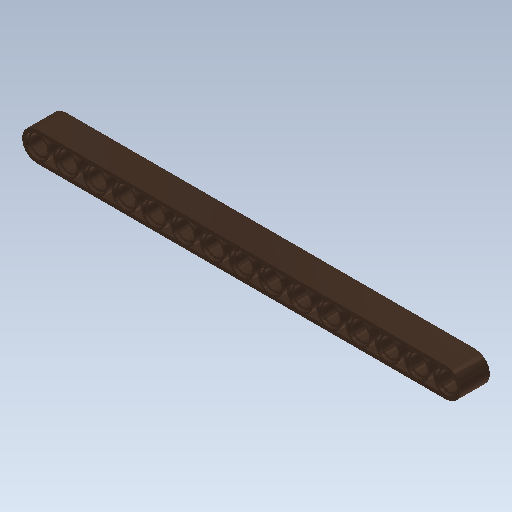
# Autodesk Inventor part: 15M Beam
Saved by Autodesk Inventor 2020 (Build 240168000, 168)
## iProperties
Created: 2014-02-10
Part Number: 15M Beam
Document SubType Name: Modeling
Designer: jleonard
Density: 8.87 g/cm^3
Material: Bronze, Cast
Appearance: Bronze - Satin
Author: jleonard
Autodesk Inventor part; units mm, degrees
ref_plane "YZ Plane" through (0, 0, 0) normal (1, 0, 0) x (0, 1, 0)
ref_plane "XZ Plane" through (0, 0, 0) normal (0, 1, 0) x (-1, 0, 0)
ref_plane "XY Plane" through (0, 0, 0) normal (0, 0, 1) x (1, 0, 0)
sketch "Sketch2" plane through (0, 0, 0) normal (0, 0, 1) x (1, 0, 0)
  arc A0 (-56, 4) -> (-56, -4) centre (-56, 0) ccw
  arc A1 (56, -4) -> (56, 4) centre (56, 0) ccw
  line L0 (-56, 4) -> (56, 4)
  line L1 (-56, -4) -> (56, -4)
  line L2 (-84, 0) -> (84, 0) projected
  line L3 (0, -5.6) -> (0, 5.6) projected
  point P0 (0, 0)
  dimension "d0" = 4
  dimension "d1" = 4
  dimension "d2" = 112
  dimension "d3" = 0
  dimension "d4" = 56
  dimension "d9" = 180
  dimension "d10" = 0
  dimension "d268" = 112
  constraints: 6 point on circle, 4 end point, 2 centre point, 2 point on line, 2 tangent
  measures "d0" radius of A0
  measures "d1" radius of A1
  measures "d2" distance of A1.centre A0.centre
  measures "d3" distance from line of A0.centre L2
  measures "d4" distance from line of A0.centre L3
  measures "d9" angle of L0 L2
  measures "d10" distance from line of L2 A1.centre
  measures "d268" distance of L1.start L1.end
extrude "Extrusion1" add sketch "Sketch2" along normal blind 8
sketch "Sketch27" plane through (0, 0, 8) normal (0, 0, 1) x (1, 0, 0)
  arc A0 (-56, 4) -> (-56, -4) centre (-56, 0) ccw projected
  circle A1 centre (-56, 0) radius 2.5
  line L0 (-84, 0) -> (84, 0) projected
  circle A2 centre (-48, 0) radius 2.5
  circle A3 centre (-40, 0) radius 2.5
  circle A4 centre (-32, 0) radius 2.5
  circle A5 centre (-24, 0) radius 2.5
  circle A6 centre (-16, 0) radius 2.5
  circle A7 centre (-8, 0) radius 2.5
  circle A8 centre (0, 0) radius 2.5
  circle A9 centre (8, 0) radius 2.5
  circle A10 centre (16, 0) radius 2.5
  circle A11 centre (24, 0) radius 2.5
  circle A12 centre (32, 0) radius 2.5
  circle A13 centre (40, 0) radius 2.5
  circle A14 centre (48, 0) radius 2.5
  circle A15 centre (56, 0) radius 2.5
  dimension "d269" = 5
  dimension "d275" = 8
  constraints: 15 centre point, 1 coincident, 1 horizontal, 28 other
  measures "d269" diameter of A1
  measures "d275" distance of A1.centre A2.centre
extrude "Extrusion26" cut sketch "Sketch27" against normal through all
sketch "Sketch28" plane through (0, 0, 8) normal (0, 0, 1) x (1, 0, 0)
  circle A0 centre (56, 0) radius 2.5 projected
  circle A1 centre (48, 0) radius 2.5 projected
  circle A2 centre (40, 0) radius 2.5 projected
  circle A3 centre (32, 0) radius 2.5 projected
  circle A4 centre (24, 0) radius 2.5 projected
  circle A5 centre (16, 0) radius 2.5 projected
  circle A6 centre (8, 0) radius 2.5 projected
  circle A7 centre (0, 0) radius 2.5 projected
  circle A8 centre (-8, 0) radius 2.5 projected
  circle A9 centre (-16, 0) radius 2.5 projected
  circle A10 centre (-24, 0) radius 2.5 projected
  circle A11 centre (-32, 0) radius 2.5 projected
  circle A12 centre (-40, 0) radius 2.5 projected
  circle A13 centre (-48, 0) radius 2.5 projected
  circle A14 centre (-56, 0) radius 2.5 projected
  arc A15 (-56, 4) -> (-56, -4) centre (-56, 0) ccw projected
  circle A16 centre (-56, 0) radius 3
  line L0 (-84, 0) -> (84, 0) projected
  circle A17 centre (-48, 0) radius 3
  circle A18 centre (-40, 0) radius 3
  circle A19 centre (-32, 0) radius 3
  circle A20 centre (-24, 0) radius 3
  circle A21 centre (-16, 0) radius 3
  circle A22 centre (-8, 0) radius 3
  circle A23 centre (0, 0) radius 3
  circle A24 centre (8, 0) radius 3
  circle A25 centre (16, 0) radius 3
  circle A26 centre (24, 0) radius 3
  circle A27 centre (32, 0) radius 3
  circle A28 centre (40, 0) radius 3
  circle A29 centre (48, 0) radius 3
  circle A30 centre (56, 0) radius 3
  dimension "d279" = 6
  dimension "d285" = 8
  constraints: 15 centre point, 1 coincident, 1 horizontal, 28 other
  measures "d279" diameter of A16
  measures "d285" distance of A16.centre A17.centre
extrude "Extrusion27" cut sketch "Sketch28" against normal blind 0.8 contours L0 A30 A0 | A0 L0 A30 | A16 L0 A14 | L0 A14 A16 | A17 L0 A13 | L0 A13 A17 | A18 L0 A12 | L0 A12 A18 | A19 L0 A11 | L0 A11 A19 | A20 L0 A10 | L0 A10 A20 | A21 L0 A9 | L0 A9 A21 | A22 L0 A8 | L0 A8 A22 | A23 L0 A7 | L0 A7 A23 | A24 L0 A6 | L0 A6 A24 | A25 L0 A5 | L0 A5 A25 | A26 L0 A4 | L0 A4 A26 | A27 L0 A3 | L0 A3 A27 | A28 L0 A2 | L0 A2 A28 | A29 L0 A1 | L0 A1 A29
sketch "Sketch29" plane through (0, 0, 0) normal (0, 0, -1) x (-1, 0, 0)
  circle A0 centre (-56, 0) radius 2.5 projected
  circle A1 centre (-48, 0) radius 2.5 projected
  circle A2 centre (-40, 0) radius 2.5 projected
  circle A3 centre (-32, 0) radius 2.5 projected
  circle A4 centre (-24, 0) radius 2.5 projected
  circle A5 centre (-16, 0) radius 2.5 projected
  circle A6 centre (-8, 0) radius 2.5 projected
  circle A7 centre (0, 0) radius 2.5 projected
  circle A8 centre (8, 0) radius 2.5 projected
  circle A9 centre (16, 0) radius 2.5 projected
  circle A10 centre (24, 0) radius 2.5 projected
  circle A11 centre (32, 0) radius 2.5 projected
  circle A12 centre (40, 0) radius 2.5 projected
  circle A13 centre (48, 0) radius 2.5 projected
  circle A14 centre (56, 0) radius 2.5 projected
  arc A15 (-56, 4) -> (-56, -4) centre (-56, 0) ccw projected
  circle A16 centre (-56, 0) radius 3
  line L0 (84, 0) -> (-84, 0) projected
  circle A17 centre (-48, 0) radius 3
  circle A18 centre (-40, 0) radius 3
  circle A19 centre (-32, 0) radius 3
  circle A20 centre (-24, 0) radius 3
  circle A21 centre (-16, 0) radius 3
  circle A22 centre (-8, 0) radius 3
  circle A23 centre (0, 0) radius 3
  circle A24 centre (8, 0) radius 3
  circle A25 centre (16, 0) radius 3
  circle A26 centre (24, 0) radius 3
  circle A27 centre (32, 0) radius 3
  circle A28 centre (40, 0) radius 3
  circle A29 centre (48, 0) radius 3
  circle A30 centre (56, 0) radius 3
  dimension "d289" = 6
  dimension "d295" = 8
  constraints: 15 centre point, 1 coincident, 1 horizontal, 28 other
  measures "d289" diameter of A16
  measures "d295" distance of A16.centre A17.centre
extrude "Extrusion28" cut sketch "Sketch29" against normal blind 0.8 contours L0 A16 A0 | A0 L0 A16 | A30 L0 A14 | L0 A14 A30 | A29 L0 A13 | L0 A13 A29 | A28 L0 A12 | L0 A12 A28 | A27 L0 A11 | L0 A11 A27 | A26 L0 A10 | L0 A10 A26 | A25 L0 A9 | L0 A9 A25 | A24 L0 A8 | L0 A8 A24 | A23 L0 A7 | L0 A7 A23 | A22 L0 A6 | L0 A6 A22 | A21 L0 A5 | L0 A5 A21 | A20 L0 A4 | L0 A4 A20 | A19 L0 A3 | L0 A3 A19 | A18 L0 A2 | L0 A2 A18 | A17 L0 A1 | L0 A1 A17
sketch "Sketch30" plane through (0, 0, 8) normal (0, 0, 1) x (1, 0, 0)
  circle A0 centre (-56, 0) radius 3 projected
  circle A1 centre (-48, 0) radius 3 projected
  arc A2 (-56, 4) -> (-56, -4) centre (-56, 0) ccw projected
  line L0 (-49.8028, 3) -> (-54.1972, 3)
  line L1 (-49.8028, -3) -> (-54.1972, -3)
  arc A3 (-54.1972, -3) -> (-54.1972, 3) centre (-56, 0) ccw
  arc A4 (-49.8028, 3) -> (-49.8028, -3) centre (-48, 0) ccw
  line L2 (-84, 0) -> (84, 0) projected
  line L3 (-41.8028, 3) -> (-46.1972, 3)
  line L4 (-41.8028, -3) -> (-46.1972, -3)
  arc A5 (-46.1972, -3) -> (-46.1972, 3) centre (-48, 0) ccw
  arc A6 (-41.8028, 3) -> (-41.8028, -3) centre (-40, 0) ccw
  line L5 (-33.8028, 3) -> (-38.1972, 3)
  line L6 (-33.8028, -3) -> (-38.1972, -3)
  arc A7 (-38.1972, -3) -> (-38.1972, 3) centre (-40, 0) ccw
  arc A8 (-33.8028, 3) -> (-33.8028, -3) centre (-32, 0) ccw
  line L7 (-25.8028, 3) -> (-30.1972, 3)
  line L8 (-25.8028, -3) -> (-30.1972, -3)
  arc A9 (-30.1972, -3) -> (-30.1972, 3) centre (-32, 0) ccw
  arc A10 (-25.8028, 3) -> (-25.8028, -3) centre (-24, 0) ccw
  line L9 (-17.8028, 3) -> (-22.1972, 3)
  line L10 (-17.8028, -3) -> (-22.1972, -3)
  arc A11 (-22.1972, -3) -> (-22.1972, 3) centre (-24, 0) ccw
  arc A12 (-17.8028, 3) -> (-17.8028, -3) centre (-16, 0) ccw
  line L11 (-9.8028, 3) -> (-14.1972, 3)
  line L12 (-9.8028, -3) -> (-14.1972, -3)
  arc A13 (-14.1972, -3) -> (-14.1972, 3) centre (-16, 0) ccw
  arc A14 (-9.8028, 3) -> (-9.8028, -3) centre (-8, 0) ccw
  line L13 (-1.8028, 3) -> (-6.1972, 3)
  line L14 (-1.8028, -3) -> (-6.1972, -3)
  arc A15 (-6.1972, -3) -> (-6.1972, 3) centre (-8, 0) ccw
  arc A16 (-1.8028, 3) -> (-1.8028, -3) centre (0, 0) ccw
  line L15 (6.1972, 3) -> (1.8028, 3)
  line L16 (6.1972, -3) -> (1.8028, -3)
  arc A17 (1.8028, -3) -> (1.8028, 3) centre (0, 0) ccw
  arc A18 (6.1972, 3) -> (6.1972, -3) centre (8, 0) ccw
  line L17 (14.1972, 3) -> (9.8028, 3)
  line L18 (14.1972, -3) -> (9.8028, -3)
  arc A19 (9.8028, -3) -> (9.8028, 3) centre (8, 0) ccw
  arc A20 (14.1972, 3) -> (14.1972, -3) centre (16, 0) ccw
  line L19 (22.1972, 3) -> (17.8028, 3)
  line L20 (22.1972, -3) -> (17.8028, -3)
  arc A21 (17.8028, -3) -> (17.8028, 3) centre (16, 0) ccw
  arc A22 (22.1972, 3) -> (22.1972, -3) centre (24, 0) ccw
  line L21 (30.1972, 3) -> (25.8028, 3)
  line L22 (30.1972, -3) -> (25.8028, -3)
  arc A23 (25.8028, -3) -> (25.8028, 3) centre (24, 0) ccw
  arc A24 (30.1972, 3) -> (30.1972, -3) centre (32, 0) ccw
  line L23 (38.1972, 3) -> (33.8028, 3)
  line L24 (38.1972, -3) -> (33.8028, -3)
  arc A25 (33.8028, -3) -> (33.8028, 3) centre (32, 0) ccw
  arc A26 (38.1972, 3) -> (38.1972, -3) centre (40, 0) ccw
  line L25 (46.1972, 3) -> (41.8028, 3)
  line L26 (46.1972, -3) -> (41.8028, -3)
  arc A27 (41.8028, -3) -> (41.8028, 3) centre (40, 0) ccw
  arc A28 (46.1972, 3) -> (46.1972, -3) centre (48, 0) ccw
  line L27 (54.1972, 3) -> (49.8028, 3)
  line L28 (54.1972, -3) -> (49.8028, -3)
  arc A29 (49.8028, -3) -> (49.8028, 3) centre (48, 0) ccw
  arc A30 (54.1972, 3) -> (54.1972, -3) centre (56, 0) ccw
  dimension "d299" = 7
  dimension "d300" = 7
  dimension "d306" = 8
  constraints: 56 end point, 56 point on circle, 28 centre point, 4 tangent, 2 coincident, 1 horizontal, 130 other
  measures "d299" diameter of A3
  measures "d300" diameter of A4
  measures "d306" distance of L0.start L3.start
extrude "Extrusion29" cut sketch "Sketch30" against normal through all contours A29 L27 A30 L2 | L2 A30 L28 A29 | A27 L25 A28 L2 | L2 A28 L26 A27 | A25 L23 A26 L2 | L2 A26 L24 A25 | A23 L21 A24 L2 | L2 A24 L22 A23 | A21 L19 A22 L2 | L2 A22 L20 A21 | A19 L17 A20 L2 | L2 A20 L18 A19 | A17 L15 A18 L2 | L2 A18 L16 A17 | A15 L13 A16 L2 | L2 A16 L14 A15 | A13 L11 A14 L2 | L2 A14 L12 A13 | A11 L9 A12 L2 | L2 A12 L10 A11 | A9 L7 A10 L2 | L2 A10 L8 A9 | A7 L5 A8 L2 | L2 A8 L6 A7 | A5 L3 A6 L2 | L2 A6 L4 A5 | A3 L0 A4 L2 | L2 A4 L1 A3
equation "\"d4\" = 0.5 * d2"
body "Solid1"
